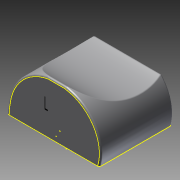
# Autodesk Inventor part: L Button
Saved by Autodesk Inventor 2012 SP1 (Build 160190100, 190)
## iProperties
Created: 2012-01-06
Part Number: L Button
Material: Default
Document SubType Name: Modeling
Designer: 133098
Density: 1 g/cm^3
Author: 133098
Autodesk Inventor part; units mm, degrees
ref_plane "YZ Plane" through (0, 0, 0) normal (1, 0, 0) x (0, 1, 0)
ref_plane "XZ Plane" through (0, 0, 0) normal (0, 1, 0) x (-1, 0, 0)
ref_plane "XY Plane" through (0, 0, 0) normal (0, 0, 1) x (1, 0, 0)
sketch "Sketch1" plane through (0, 0, 0) normal (0, 0, 1) x (1, 0, 0)
  arc A0 (1.9236, 10.6222) -> (-13.589, 0) centre (-0.9971, -1.7508) ccw
  arc A1 (-13.589, 0) -> (-13.9148, -3.0469) centre (1.6936, -3.175) ccw
  line L0 (0, -3.0469) -> (-13.9148, -3.0469)
  line L1 (0, -3.0469) -> (10.3561, -3.0469)
  arc A2 (10.3561, -3.0469) -> (1.9236, 10.6222) centre (0, 0) ccw
  constraints: 6 point on circle, 4 end point, 3 centre point, 1 collinear
extrude "Extrusion1" add sketch "Sketch1" along normal blind 19.05
fillet "Fillet1" radius 0.4445 6 edges at (-8.1798, 8.7388, 19.05) (9.1874, 5.6677, 19.05) (-8.1798, 8.7388, 0) (-13.8268, -1.5154, 0) (-13.8268, -1.5154, 19.05) (9.1874, 5.6677, 0)
sketch "Sketch3" plane through (0, 0, 0) normal (1, 0, 0) x (0, 1, 0)
  arc A0 (6.7945, 9.525) -> (11.1125, 19.05) centre (26.5462, 6.3122) ccw
  circle A1 centre (26.5462, 6.3122) radius 20.0113
  point P0 (0, 0)
  constraints: 2 point on circle, 1 centre point, 1 coincident, 3 other
extrude "Extrusion3" cut sketch "Sketch3" along normal mid plane 25.4
fillet "Fillet2" radius 0.381 9 edges at (7.5437, 7.5182, 0.1164) (8.1516, 7.077, 10.9383) (-9.4831, 7.5186, 0.1152) (-10.0835, 7.1407, 11.1988) (-1.6514, 10.9039, 18.793) (0.6521, 10.8413, 18.7141) (1.6051, 10.6931, 18.5241) (-4.4952, 7.5565, 0) (3.5367, 7.5565, 0)
sketch "Sketch4" plane through (0, 0, 19.05) normal (0, 0, 1) x (1, 0, 0)
  line L0 (-3.168, 10.3242) -> (1.1738, 10.3242) projected
  arc A0 (-3.168, 10.3242) -> (-13.1508, -0.0759) centre (-0.9971, -1.7508) ccw projected
  arc A1 (-13.1508, -0.0759) -> (-13.4703, -3.0469) centre (1.6936, -3.175) ccw projected
  line L1 (9.8919, -3.0469) -> (-13.4703, -3.0469) projected
  arc A2 (9.8919, -3.0469) -> (1.8329, 10.1869) centre (0, 0) ccw projected
  arc A3 (1.8329, 10.1869) -> (1.1738, 10.3242) centre (-0.9971, -1.7508) ccw projected
  line L2 (-4.2322, 5.918) -> (4.1137, 5.918) construction
  line L3 (4.1137, 5.918) -> (4.1137, -1.6056) construction
  line L4 (4.1137, -1.6056) -> (-4.2322, -1.6056) construction
  line L5 (-4.2322, -1.6056) -> (-4.2322, 5.918) construction
  constraints: 2 other
sketch "Sketch5" plane through (-13.4703, -3.0469, 0) normal (0, -1, 0) x (1, 0, 0)
  arc A0 (23.8264, 0.4445) -> (23.3622, 0) centre (23.3622, 0) ccw projected
  line L0 (23.8264, 0.4445) -> (23.8264, 18.6055) projected
  arc A1 (23.3622, 19.05) -> (23.8264, 18.6055) centre (23.8264, 18.6055) ccw projected
  line L1 (23.3622, 19.05) -> (0, 19.05) projected
  arc A2 (-0.4445, 18.6055) -> (0, 19.05) centre (0, 19.05) ccw projected
  line L2 (-0.4445, 0.4445) -> (-0.4445, 18.6055) projected
  arc A3 (0, 0) -> (-0.4445, 0.4445) centre (-0.4445, 0.4445) ccw projected
  line L3 (23.3622, 0) -> (0, 0) projected
  point P0 (13.4703, 0)
  constraints: 4 other
body "Solid1"
